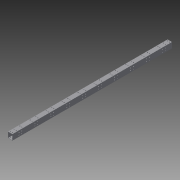
# Autodesk Inventor part: Part1
Saved by Autodesk Inventor 2015 SP1 (Build 190203100, 203)
## iProperties
Created: 2015-03-28
Part Number: Part1
Material: Generic
Document SubType Name: Modeling
Designer: Cyril
Density: 1 g/cm^3
Appearance: Default
Author: Cyril
Autodesk Inventor part; units mm, degrees
ref_plane "YZ Plane" through (0, 0, 0) normal (1, 0, 0) x (0, 1, 0)
ref_plane "XZ Plane" through (0, 0, 0) normal (0, 1, 0) x (-1, 0, 0)
ref_plane "XY Plane" through (0, 0, 0) normal (0, 0, 1) x (1, 0, 0)
sketch "Sketch2" plane through (0, 0, 0) normal (0, 0, 1) x (1, 0, 0)
  line L0 (-18, -23) -> (18, -23)
  line L1 (18, -23) -> (18, 23)
  line L2 (18, 23) -> (-18, 23)
  line L3 (-18, 23) -> (-18, -23)
  line L4 (-18, -22.5) -> (18, 22.5) construction
  line L5 (18, -23) -> (-15.1101, 19.3073) construction
  line L6 (-20, -25) -> (20, -25)
  line L7 (20, -25) -> (20, 25)
  line L8 (20, 25) -> (-20, 25)
  line L9 (-20, 25) -> (-20, -25)
  line L10 (-20, -25) -> (20, 25) construction
  line L11 (20, -25) -> (-20, 25) construction
  point P0 (0, 0)
  dimension "d0" = 40
  dimension "d1" = 50
  dimension "d3" = 2
  dimension "d6" = 2
  dimension "d7" = 2
  dimension "d8" = 2
  constraints: 24 end point, 4 parallel, 3 midpoint, 2 horizontal, 2 perpendicular, 2 point on line
  measures "d0" distance of L7.end L8.end
  measures "d1" distance of L8.end L6.start
  measures "d3" distance between parallel lines of L9 L3
  measures "d6" distance between parallel lines of L8 L2
  measures "d7" distance between parallel lines of L7 L1
  measures "d8" distance between parallel lines of L6 L0
extrude "Extrusion1" add sketch "Sketch2" along normal mid plane 1430
sketch "Sketch3" plane through (-20, -25, 715) normal (-1, 0, 0) x (0, 0, 1)
  circle A0 centre (-84, 33) radius 3.5
  circle A1 centre (-59, 33) radius 3.5
  circle A2 centre (-84, 13) radius 3.5
  circle A3 centre (-59, 13) radius 3.5
  line L0 (0, 0) -> (-1430, 0) projected
  line L1 (0, 50) -> (0, 0) projected
  circle A4 centre (-227, 33) radius 3.5
  circle A5 centre (-202, 33) radius 3.5
  circle A6 centre (-227, 13) radius 3.5
  circle A7 centre (-202, 13) radius 3.5
  circle A8 centre (-370, 33) radius 3.5
  circle A9 centre (-345, 33) radius 3.5
  circle A10 centre (-370, 13) radius 3.5
  circle A11 centre (-345, 13) radius 3.5
  circle A12 centre (-513, 33) radius 3.5
  circle A13 centre (-488, 33) radius 3.5
  circle A14 centre (-513, 13) radius 3.5
  circle A15 centre (-488, 13) radius 3.5
  circle A16 centre (-656, 33) radius 3.5
  circle A17 centre (-631, 33) radius 3.5
  circle A18 centre (-656, 13) radius 3.5
  circle A19 centre (-631, 13) radius 3.5
  circle A20 centre (-799, 33) radius 3.5
  circle A21 centre (-774, 33) radius 3.5
  circle A22 centre (-799, 13) radius 3.5
  circle A23 centre (-774, 13) radius 3.5
  circle A24 centre (-942, 33) radius 3.5
  circle A25 centre (-917, 33) radius 3.5
  circle A26 centre (-942, 13) radius 3.5
  circle A27 centre (-917, 13) radius 3.5
  circle A28 centre (-1085, 33) radius 3.5
  circle A29 centre (-1060, 33) radius 3.5
  circle A30 centre (-1085, 13) radius 3.5
  circle A31 centre (-1060, 13) radius 3.5
  circle A32 centre (-1228, 33) radius 3.5
  circle A33 centre (-1203, 33) radius 3.5
  circle A34 centre (-1228, 13) radius 3.5
  circle A35 centre (-1203, 13) radius 3.5
  circle A36 centre (-1371, 33) radius 3.5
  circle A37 centre (-1346, 33) radius 3.5
  circle A38 centre (-1371, 13) radius 3.5
  circle A39 centre (-1346, 13) radius 3.5
  point P0 (-715, 25)
  dimension "d9" = 7
  dimension "d10" = 25
  dimension "d11" = 20
  dimension "d12" = 13
  dimension "d13" = 59
  dimension "d16" = 143
  constraints: 40 centre point, 3 equal radius, 2 horizontal alignment, 2 vertical alignment, 1 horizontal, 72 other
  measures "d9" diameter of A0
  measures "d10" distance of A1.centre A0.centre
  measures "d11" distance of A2.centre A0.centre
  measures "d12" distance from line of L0 A3.centre
  measures "d13" distance from line of A3.centre L1
  measures "d16" distance of A0.centre A4.centre
extrude "Extrusion2" cut sketch "Sketch3" against normal through all
sketch "Sketch4" plane through (-20, 25, 715) normal (0, 1, 0) x (1, 0, 0)
  circle A0 centre (11, 12.5) radius 3.5
  circle A1 centre (29, 12.5) radius 3.5
  line L0 (40, 0) -> (0, 0) projected
  line L1 (0, 0) -> (40, 0) projected
  line L2 (20, 0) -> (20, 1430) construction
  line L3 (0, 1430) -> (40, 1430) projected
  circle A2 centre (11, 1417.5) radius 3.5
  circle A3 centre (29, 1417.5) radius 3.5
  point P0 (20, 715)
  dimension "d23" = 7
  dimension "d24" = 12.5
  dimension "d25" = 18
  dimension "d26" = 12.5
  constraints: 4 centre point, 3 equal radius, 2 end point, 2 horizontal alignment, 2 midpoint, 2 vertical alignment, 1 other
  measures "d23" diameter of A0
  measures "d24" distance from line of L0 A0.centre
  measures "d25" distance of A1.centre A0.centre
  measures "d26" distance from line of L3 A2.centre
extrude "Extrusion3" cut sketch "Sketch4" against normal through all
sketch "Sketch5" plane through (-20, 25, 715) normal (0, 1, 0) x (1, 0, 0)
  circle A0 centre (10, 96.5) radius 3.5
  circle A1 centre (28, 96.5) radius 3.5
  circle A2 centre (28, 46.5) radius 3.5
  circle A3 centre (10, 46.5) radius 3.5
  line L0 (0, 1430) -> (0, 0) projected
  line L1 (40, 0) -> (0, 0) projected
  circle A4 centre (10, 239.5) radius 3.5
  circle A5 centre (28, 239.5) radius 3.5
  circle A6 centre (28, 189.5) radius 3.5
  circle A7 centre (10, 189.5) radius 3.5
  circle A8 centre (10, 382.5) radius 3.5
  circle A9 centre (28, 382.5) radius 3.5
  circle A10 centre (28, 332.5) radius 3.5
  circle A11 centre (10, 332.5) radius 3.5
  circle A12 centre (10, 525.5) radius 3.5
  circle A13 centre (28, 525.5) radius 3.5
  circle A14 centre (28, 475.5) radius 3.5
  circle A15 centre (10, 475.5) radius 3.5
  circle A16 centre (10, 668.5) radius 3.5
  circle A17 centre (28, 668.5) radius 3.5
  circle A18 centre (28, 618.5) radius 3.5
  circle A19 centre (10, 618.5) radius 3.5
  circle A20 centre (10, 811.5) radius 3.5
  circle A21 centre (28, 811.5) radius 3.5
  circle A22 centre (28, 761.5) radius 3.5
  circle A23 centre (10, 761.5) radius 3.5
  circle A24 centre (10, 954.5) radius 3.5
  circle A25 centre (28, 954.5) radius 3.5
  circle A26 centre (28, 904.5) radius 3.5
  circle A27 centre (10, 904.5) radius 3.5
  circle A28 centre (10, 1097.5) radius 3.5
  circle A29 centre (28, 1097.5) radius 3.5
  circle A30 centre (28, 1047.5) radius 3.5
  circle A31 centre (10, 1047.5) radius 3.5
  circle A32 centre (10, 1240.5) radius 3.5
  circle A33 centre (28, 1240.5) radius 3.5
  circle A34 centre (28, 1190.5) radius 3.5
  circle A35 centre (10, 1190.5) radius 3.5
  circle A36 centre (10, 1383.5) radius 3.5
  circle A37 centre (28, 1383.5) radius 3.5
  circle A38 centre (28, 1333.5) radius 3.5
  circle A39 centre (10, 1333.5) radius 3.5
  point P0 (20, 715)
  dimension "d29" = 10
  dimension "d30" = 18
  dimension "d31" = 46.5
  dimension "d32" = 7
  dimension "d33" = 50
  dimension "d36" = 143
  constraints: 40 centre point, 3 equal radius, 2 horizontal alignment, 2 vertical alignment, 1 vertical, 72 other
  measures "d29" distance from line of L0 A3.centre
  measures "d30" distance of A2.centre A3.centre
  measures "d31" distance from line of A3.centre L1
  measures "d32" diameter of A0
  measures "d33" distance of A0.centre A3.centre
  measures "d36" distance of A0.centre A4.centre
extrude "Extrusion4" cut sketch "Sketch5" against normal through all
equation "\"d6\" = d3"
equation "\"d7\" = d3"
equation "\"d26\" = d24"
body "Solid1"
